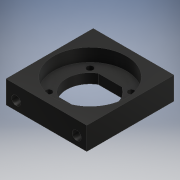
# Autodesk Inventor part: MotorMountv2
Saved by Autodesk Inventor 2017 (Build 210142000, 142)
## iProperties
Created: 2019-06-10
Part Number: MotorMountv2
Material: Generic
Document SubType Name: Modeling
Designer: cresswnd
Density: 1 g/cm^3
Appearance: Glossy - Black
Author: cresswnd
Autodesk Inventor part; units mm, degrees
ref_plane "YZ Plane" through (0, 0, 0) normal (1, 0, 0) x (0, 1, 0)
ref_plane "XZ Plane" through (0, 0, 0) normal (0, 1, 0) x (-1, 0, 0)
ref_plane "XY Plane" through (0, 0, 0) normal (0, 0, 1) x (1, 0, 0)
sketch "Sketch1" plane through (0, 0, 0) normal (0, 0, 1) x (1, 0, 0)
  circle A0 centre (-6.364, 6.364) radius 1
  circle A1 centre (6.364, 6.364) radius 1
  circle A2 centre (6.364, -6.364) radius 1
  circle A3 centre (-6.364, -6.364) radius 1
  line L0 (-12.5, 13.5) -> (12.5, 13.5)
  line L1 (12.5, 13.5) -> (12.5, -13.5)
  line L2 (12.5, -13.5) -> (-12.5, -13.5)
  line L3 (-12.5, -13.5) -> (-12.5, 13.5)
  line L4 (0, 13.5) -> (-9.375, 13.5) construction
  line L5 (0, 6) -> (0, -6) construction
  line L6 (0, 6) -> (0, 6.25) construction
  line L7 (0, -6) -> (0, -6.25) construction
  line L8 (3.9, -6.25) -> (-8.1, -6.25) construction
  line L9 (4.1, 6.25) -> (-8.9, 6.25) construction
  line L10 (0, 6) -> (3.6056, 6) construction
  line L11 (0, 6.25) -> (3.7, 6.25) construction
  line L12 (3.7, 6.25) -> (-3.7, 6.25)
  line L13 (3.7, -6.25) -> (-3.7, -6.25)
  line L14 (0, 0) -> (7.25, 0) construction
  line L15 (0, 0) -> (-7.25, 0)
  arc A4 (-3.7, 6.25) -> (-3.7, -6.25) centre (0.0268, 0) ccw
  arc A5 (3.7, -6.25) -> (3.7, 6.25) centre (-0.0268, 0) ccw
  point P0 (12.5, 0)
  point P1 (0, -6.25)
  dimension "d0" = 27
  dimension "d1" = 25
  dimension "d2" = 9.375
  dimension "d3" = 12
  dimension "d4" = 0.25
  dimension "d5" = 0.25
  dimension "d6" = 3.6056
  dimension "d7" = 3.7
  dimension "d8" = 7.4
  dimension "d10" = 7.4
  dimension "d11" = 7.25
  dimension "d25" = 7.25
  constraints: 32 end point, 6 centre point, 6 point on circle, 5 horizontal, 5 point on line, 4 midpoint, 2 parallel, 2 vertical, 2 vertical alignment, 1 horizontal alignment, 1 perpendicular
  measures "d0" distance of L0.end L1.end
  measures "d1" distance of L0.start L0.end
  measures "d2" distance of L4.start L4.end
  measures "d3" distance of L5.start L5.end
  measures "d4" distance of L5.start L6.end
  measures "d5" distance of L5.end L7.end
  measures "d6" distance of L5.start L10.end
  measures "d7" distance of L6.end L11.end
  measures "d8" distance of L11.end L12.end
  measures "d10" distance of L13.start L13.end
  measures "d11" distance of L14.start L14.end
  measures "d25" distance of L14.start L15.end
extrude "Extrusion1" add sketch "Sketch1" along normal blind 3
sketch "Sketch2" plane through (0, 0, 3) normal (0, 0, 1) x (1, 0, 0)
  line L0 (3.7, -6.25) -> (-3.7, -6.25) projected
  line L1 (-3.7, 6.25) -> (3.7, 6.25) projected
  circle A0 centre (-6.364, -6.364) radius 1 projected
  circle A1 centre (6.364, -6.364) radius 1 projected
  circle A2 centre (6.364, 6.364) radius 1 projected
  circle A3 centre (-6.364, 6.364) radius 1 projected
  line L2 (12.5, 13.5) -> (-12.5, 13.5) projected
  line L3 (-12.5, 13.5) -> (-12.5, -13.5) projected
  line L4 (-12.5, -13.5) -> (12.5, -13.5) projected
  line L5 (12.5, -13.5) -> (12.5, 13.5) projected
  circle A4 centre (0, 0) radius 11
  arc A5 (3.7, -6.25) -> (3.7, 6.25) centre (-0.0268, 0) ccw projected
  arc A6 (-3.7, 6.25) -> (-3.7, -6.25) centre (0.0268, 0) ccw projected
  dimension "d14" = 22
  constraints: 1 centre point, 1 coincident
  measures "d14" diameter of A4
extrude "Extrusion2" add sketch "Sketch2" along normal blind 2.5 contours L5 L4 L3 L2
sketch "Sketch3" plane through (-12.5, 13.5, 0) normal (0, 1, 0) x (1, 0, 0)
  line L0 (0, 0) -> (25, 0) projected
  line L1 (0, 0) -> (0, -5.5) projected
  line L2 (25, -5.5) -> (0, -5.5) projected
  line L3 (25, 0) -> (25, -5.5) projected
  line L4 (12.5, 0) -> (12.5, -5.5) construction
  line L5 (25, -5.5) -> (0, -5.5) construction
  line L6 (12.5, 0) -> (12.5, -2.75) construction
  line L7 (12.5, -2.75) -> (3.125, -2.75) construction
  line L8 (12.5, -2.75) -> (21.875, -2.75) construction
  circle A0 centre (3.125, -2.75) radius 1.4
  circle A1 centre (21.875, -2.75) radius 1.4
  dimension "d17" = 2.75
  dimension "d18" = 9.375
  dimension "d19" = 180
  dimension "d20" = 2.8
  dimension "d21" = 2.8
  constraints: 8 end point, 2 centre point, 2 coincident, 2 horizontal, 2 midpoint, 1 collinear
  measures "d17" distance of L4.start L6.end
  measures "d18" distance of L6.end L7.end
  measures "d19" angle of L7 L8
  measures "d20" diameter of A0
  measures "d21" diameter of A1
extrude "Extrusion3" cut sketch "Sketch3" against normal blind 5.5 contours A0 | A1
mirror "Mirror1" about plane through (0, 0, 0) normal (0, 1, 0) of "Extrusion3"
sketch "Sketch4" plane through (0, 0, 5.5) normal (0, 0, 1) x (1, 0, 0)
  circle A0 centre (0, 0) radius 11 projected
  line L0 (12.5, 13.5) -> (-12.5, 13.5) projected
  line L1 (-12.5, 13.5) -> (-12.5, -13.5) projected
  line L2 (-12.5, -13.5) -> (12.5, -13.5) projected
  line L3 (12.5, -13.5) -> (12.5, 13.5) projected
extrude "Extrusion4" add sketch "Sketch4" along normal blind 1.5
sketch "Sketch5" plane through (0, 0, 7) normal (0, 0, 1) x (1, 0, 0)
  circle A0 centre (0, 0) radius 11.25
  circle A1 centre (0, 0) radius 11 projected
  dimension "d28" = 22.5
  constraints: 1 centre point, 1 coincident
  measures "d28" diameter of A0
extrude "Extrusion5" cut sketch "Sketch5" against normal up to surface (4 mm away)
body "Solid1"
